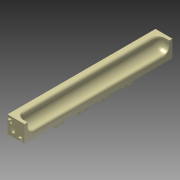
# Autodesk Inventor part: Pillar2
Saved by Autodesk Inventor 2015 (Build 190159000, 159)
## iProperties
Created: 2015-04-20
Part Number: Pillar2
Material: NylonD2W
Document SubType Name: Modeling
Designer: Akovo_000
Density: 1.13 g/cm^3
Appearance: Nylon 6
Mass: 21.3766 g
Surface Area: 162.248 cm^2
Volume: 18.9174 cm^3
Author: Akovo_000
Autodesk Inventor part; units mm, degrees
ref_plane "YZ Plane" through (0, 0, 0) normal (1, 0, 0) x (0, 1, 0)
ref_plane "XZ Plane" through (0, 0, 0) normal (0, 1, 0) x (-1, 0, 0)
ref_plane "XY Plane" through (0, 0, 0) normal (0, 0, 1) x (1, 0, 0)
sketch "Sketch1" plane through (0, 0, 0) normal (0, 1, 0) x (-1, 0, 0)
  line L0 (16, 16) -> (7.6667, 16)
  line L1 (0, 16) -> (0, 8.3333)
  line L2 (16, 16) -> (16, 14)
  line L3 (16, 14) -> (12, 14)
  line L4 (16, 12) -> (16, 7.6667)
  line L5 (0, 0) -> (2, 0)
  line L6 (2, 0) -> (2, 4)
  line L7 (2, 4) -> (4, 4)
  line L8 (4, 0) -> (8.3333, 0)
  circle A0 centre (11, 5) radius 2
  line L9 (12, 10) -> (14, 10)
  line L10 (14, 10) -> (14, 12)
  line L11 (14, 12) -> (16, 12)
  line L12 (12, 10) -> (12, 12)
  line L13 (4, 0) -> (4, 2)
  line L14 (4, 2) -> (6, 2)
  line L15 (6, 2) -> (6, 4)
  line L16 (4, 4) -> (6, 4)
  line L17 (12, 12) -> (12, 14)
  line L18 (7.6667, 16) -> (0, 16)
  line L19 (0, 8.3333) -> (0, 0)
  line L20 (8.3333, 0) -> (16, 0)
  line L21 (16, 7.6667) -> (16, 0)
  line L22 (11, 5) -> (16, 5) construction
  line L23 (11, 5) -> (11, 0) construction
  line L24 (16, 10) -> (6, 10) construction
  line L25 (6, 0) -> (6, 10) construction
  line L26 (6, 10) -> (0, 10) construction
  line L27 (6, 10) -> (6, 16) construction
  line L28 (11, 5) -> (11, 10) construction
  line L29 (11, 5) -> (6, 5) construction
  dimension "d0" = 2
  dimension "d3" = 2
  dimension "d7" = 4
  dimension "d13" = 2
  dimension "d85" = 4
  dimension "d91" = 16
  dimension "d115" = 0
  dimension "d116" = 5
  constraints: 60 end point, 17 perpendicular, 14 equal length, 7 point on line, 6 horizontal, 6 vertical, 4 collinear, 2 midpoint, 1 centre point, 1 parallel
  measures "d0" distance of L2.end L4.start
  measures "d3" distance between parallel lines of L3 L0
  measures "d7" diameter of A0
  measures "d13" distance of L9.start L12.end
  measures "d85" distance of L3.end L2.end
  measures "d91" distance of L0.start L20.end
  measures "d115" distance between parallel lines of L25 L15
  measures "d116" distance from line of L22.start L15
extrude "Attachment Bas" add sketch "Sketch1" along normal blind 3
sketch "Sketch9" plane through (0, 3, 0) normal (0, 1, 0) x (1, 0, 0)
  line L0 (-16, -14) -> (-12, -14)
  line L1 (-12, -14) -> (-12, -10)
  line L2 (-12, -10) -> (-14, -10)
  line L3 (-14, -10) -> (-12, -10) projected
  line L4 (-14, -10) -> (-14, -12)
  line L5 (-14, -12) -> (-16, -12)
  line L6 (-16, -12) -> (-14, -12) projected
  line L7 (-16, -12) -> (-16, -5)
  line L8 (-16, 0) -> (-16, -12) projected
  line L9 (-16, 0) -> (-11, 0) construction
  line L10 (-4, 0) -> (-4, -2)
  line L11 (-4, -2) -> (-6, -2)
  line L12 (-6, -2) -> (-6, -4)
  line L13 (-6, -4) -> (-6, -2) projected
  line L14 (-6, -4) -> (-2, -4)
  line L15 (-2, -4) -> (-2, 0)
  line L16 (-2, 0) -> (-2, -4) projected
  line L17 (-2, 0) -> (0, 0)
  line L18 (0, 0) -> (-2, 0) projected
  line L19 (0, 0) -> (0, -4)
  line L20 (0, -16) -> (-12, -16) construction
  line L21 (-16, -16) -> (-16, -14)
  line L22 (-12, -14) -> (-16, -14) projected
  circle A0 centre (-11, -5) radius 2 projected
  arc A1 (-11, 0) -> (-16, -5) centre (-11, -5) ccw
  line L23 (-4, 0) -> (-16, 0) construction
  line L24 (-16, -5) -> (-16, 0) construction
  line L25 (-11, 0) -> (-4, 0)
  line L26 (-12, -16) -> (-16, -16)
  line L27 (0, -4) -> (0, -16) construction
  line L28 (0, -16) -> (0, 0) projected
  line L29 (-2, -4) -> (-6, -4) projected
  line L30 (-16, -16) -> (0, -16) projected
  circle A2 centre (-11, -5) radius 2 projected
  line L31 (-14.5355, -1.4645) -> (-12.4142, -3.5858) construction
  line L32 (-11, -5) -> (-9.5858, -6.4142) construction
  line L33 (-12, -14) -> (-9, -14) construction
  line L34 (-12, -10) -> (-12, -14) projected
  line L35 (-2, -4) -> (-2, -7) construction
  line L36 (-2, -7) -> (-2, -14) construction
  line L37 (-2, -14) -> (-9.7838, -14) construction
  line L38 (-9.5858, -6.4142) -> (-7.4645, -8.5355) construction
  line L39 (-12.4142, -3.5858) -> (-11, -5) construction
  arc A3 (-7.4645, -8.5355) -> (-9.725, -13.7869) centre (-2, -14) ccw
  arc A4 (-2.2131, -6.275) -> (-7.4645, -8.5355) centre (-2, -14) ccw
  arc A5 (-2.2131, -6.275) -> (0, -4) centre (-2.2759, -4) ccw
  arc A6 (-12, -16) -> (-9.725, -13.7869) centre (-12, -13.7241) ccw
  constraints: 56 end point, 19 perpendicular, 14 collinear, 13 point on circle, 7 tangent, 5 centre point, 5 coincident, 3 equal length, 3 point on line, 2 line through centre, 1 equal radius, 1 horizontal
extrude "curvedpart" add sketch "Sketch9" along normal blind 15 contours L0 L1 L2 L4 L5 L7 A1 L25 L10 L11 L12 L14 L15 L17 L19 A5 A4 A3 A6 L26 L21
sketch "Sketch2" plane through (0, 18, 0) normal (0, 1, 0) x (1, 0, 0)
  line L0 (0, 0) -> (-2, 0)
  line L1 (0, 0) -> (-2, 0) projected
  line L2 (-2, 0) -> (-2, -4)
  line L3 (-2, 0) -> (-2, -4) projected
  line L4 (-2, -4) -> (-6, -4)
  line L5 (-2, -4) -> (-6, -4) projected
  line L6 (-6, -4) -> (-6, -2)
  line L7 (-6, -4) -> (-6, -2) projected
  line L8 (-6, -2) -> (-4, -2)
  line L9 (-6, -2) -> (-4, -2) projected
  line L10 (-4, -2) -> (-4, 0)
  line L11 (-4, -2) -> (-4, 0) projected
  arc A0 (-11, 0) -> (-16, -5) centre (-11, -5) ccw projected
  arc A1 (-11, 0) -> (-16, -5) centre (-11, -5) ccw
  line L12 (-16, -5) -> (-16, -12)
  line L13 (-16, -12) -> (-14, -12)
  line L14 (-16, -12) -> (-14, -12) projected
  line L15 (-12, -10) -> (-12, -14)
  line L16 (-12, -14) -> (-16, -14)
  line L17 (-16, -14) -> (-16, -16)
  line L18 (0, -16) -> (0, 0) projected
  line L19 (-6, -4) -> (-12, -10) construction
  line L20 (-12, -10) -> (-14, -10)
  line L21 (-14, -11) -> (-12, -11) projected
  line L22 (-14, -10) -> (-14, -12)
  line L23 (-14, -12) -> (-14, -10) projected
  line L24 (0, 0) -> (0, -4)
  line L25 (-4, 0) -> (-11, 0)
  line L26 (-4, 0) -> (-16, 0) projected
  line L27 (-9.954, -1.0963) -> (-7.0963, -3.954)
  line L28 (-7.0963, -3.954) -> (-8.1423, -7.8577)
  line L29 (-8.1423, -7.8577) -> (-12.046, -8.9037)
  line L30 (-12.046, -8.9037) -> (-14.9037, -6.046)
  line L31 (-14.9037, -6.046) -> (-13.8577, -2.1423)
  line L32 (-13.8577, -2.1423) -> (-9.954, -1.0963)
  arc A2 (-2.2131, -6.275) -> (-9.725, -13.7869) centre (-2, -14) ccw
  arc A3 (-2.2131, -6.275) -> (0, -4) centre (-2.2759, -4) ccw
  arc A4 (-12, -16) -> (-9.725, -13.7869) centre (-12, -13.7241) ccw
  line L33 (-12, -16) -> (-16, -16)
  line L34 (-16, -16) -> (0, -16) projected
  dimension "d103" = 7
  constraints: 46 end point, 10 collinear, 8 point on circle, 4 centre point, 3 perpendicular, 3 tangent, 3 vertical, 2 coincident, 1 parallel, 13 other
  measures "d103" distance between parallel lines of L27 L30
extrude "BossForNut" add sketch "Sketch2" along normal blind 3 contours L18 A3 A2 A4 L33 L17 L16 L15 L20 L22 L13 L12 A0 L25 L10 L8 L6 L4 L2 L0
sketch "Sketch3" plane through (0, 21, 0) normal (0, 1, 0) x (1, 0, 0)
  line L0 (-16, -5) -> (-16, -6.9497)
  arc A0 (-11, 0) -> (-16, -5) centre (-11, -5) ccw projected
  line L1 (-16, -5) -> (-16, -12) projected
  line L2 (-16, -12) -> (-14, -12)
  line L3 (-14, -12) -> (-14, -10)
  line L4 (-14, -12) -> (-14, -10) projected
  line L5 (-14, -10) -> (-12, -10)
  line L6 (-12, -10) -> (-12, -14)
  line L7 (-12, -14) -> (-16, -14)
  line L8 (-16, -14) -> (-16, -16) projected
  line L9 (-16, -14) -> (-16, -16)
  arc A1 (-11, 0) -> (-11.05, -0.0003) centre (-11, -5) ccw
  line L10 (0, -4) -> (0, 0)
  line L11 (0, -4) -> (0, 0) projected
  line L12 (0, 0) -> (-2, 0)
  line L13 (0, 0) -> (-2, 0) projected
  line L14 (-2, 0) -> (-2, -4)
  line L15 (-2, -4) -> (-6, -4)
  line L16 (-2, -4) -> (-6, -4) projected
  line L17 (-6, -4) -> (-6, -2)
  line L18 (-6, -2) -> (-4, -2)
  line L19 (-6, -2) -> (-4, -2) projected
  line L20 (-4, -2) -> (-4, 0)
  line L21 (-4, 0) -> (-11, 0)
  line L22 (-4, 0) -> (-11, 0) projected
  line L23 (-8.1423, -7.8577) -> (-12.046, -8.9037)
  line L24 (-12.046, -8.9037) -> (-8.1423, -7.8577) projected
  line L25 (-12.046, -8.9037) -> (-14.9037, -6.046)
  line L26 (-14.9037, -6.046) -> (-13.8577, -2.1423) construction
  line L27 (-14.9037, -6.046) -> (-13.8577, -2.1423) projected
  line L28 (-13.8577, -2.1423) -> (-9.954, -1.0963) construction
  line L29 (-13.8577, -2.1423) -> (-9.954, -1.0963) construction
  line L30 (-9.954, -1.0963) -> (-7.0963, -3.954)
  line L31 (-7.0963, -3.954) -> (-8.1423, -7.8577)
  line L32 (-12.046, -8.9037) -> (-14.9037, -6.046) projected
  line L33 (-9.954, -1.0963) -> (-7.0963, -3.954) projected
  arc A2 (-2.2131, -6.275) -> (0, -4) centre (-2.2759, -4) ccw
  line L34 (-12, -16) -> (-16, -16)
  line L35 (-16, -16) -> (-12, -16) projected
  arc A3 (-12, -16) -> (-9.725, -13.7869) centre (-12, -13.7241) ccw
  arc A4 (-2.2131, -6.275) -> (-9.725, -13.7869) centre (-2, -14) ccw
  line L36 (-9.954, -1.0963) -> (-11.05, -0.0003)
  line L37 (-14.9037, -6.046) -> (-15.9997, -4.95)
  arc A5 (-15.9997, -4.95) -> (-16, -5) centre (-11, -5) ccw
  arc A6 (-11.05, -0.0003) -> (-15.9997, -4.95) centre (-11, -5) ccw construction
  line L38 (-16, -6.9497) -> (-16, -12)
  point P0 (-9.0503, 0)
  constraints: 50 end point, 15 collinear, 15 point on circle, 8 perpendicular, 6 centre point, 6 tangent, 2 parallel, 2 point on line, 1 coincident
extrude "NutInserter" add sketch "Sketch3" along normal blind 5 contours A0 L37 L25 L23 L31 L30 L36 L21 L20 L18 L17 L15 L14 L12 L10 A2 A4 A3 L34 L8 L7 L6 L5 L3 L2 L1 L0
sketch "Sketch4" plane through (0, 26, 0) normal (0, 1, 0) x (1, 0, 0)
  line L0 (-12, -10) -> (-14, -10)
  line L1 (-14, -10) -> (-12, -10) projected
  line L2 (-14, -10) -> (-14, -12)
  line L3 (-14, -12) -> (-14, -10) projected
  line L4 (-14, -12) -> (-16, -12)
  line L5 (-16, -12) -> (-14, -12) projected
  line L6 (-16, -12) -> (-16, -5)
  line L7 (-16, -5) -> (-16, -12) projected
  line L8 (-12, -10) -> (-12, -14)
  line L9 (-12, -14) -> (-16, -14)
  line L10 (-16, -14) -> (-16, -16)
  line L11 (-16, -14) -> (-16, -16) projected
  line L12 (-16, -16) -> (-12, -16)
  line L13 (-11, 0) -> (-4, 0)
  line L14 (-4, 0) -> (-11, 0) projected
  line L15 (-4, 0) -> (-4, -2)
  line L16 (-4, -2) -> (-6, -2)
  line L17 (-6, -2) -> (-4, -2) projected
  line L18 (-6, -2) -> (-6, -4)
  line L19 (-6, -4) -> (-2, -4)
  line L20 (-2, -4) -> (-6, -4) projected
  line L21 (-2, -4) -> (-2, 0)
  line L22 (-2, 0) -> (0, 0)
  line L23 (0, 0) -> (-2, 0) projected
  line L24 (0, 0) -> (0, -4)
  arc A0 (-11, 0) -> (-16, -5) centre (-11, -5) ccw
  arc A1 (-2.2131, -6.275) -> (0, -4) centre (-2.2759, -4) ccw
  arc A2 (-2.2131, -6.275) -> (-9.725, -13.7869) centre (-2, -14) ccw
  arc A3 (-12, -16) -> (-9.725, -13.7869) centre (-12, -13.7241) ccw
  circle A4 centre (-11, -5) radius 3
  point P0 (-11.5, -5.5)
  dimension "d130" = 6
  constraints: 32 end point, 9 collinear, 8 point on circle, 6 perpendicular, 5 centre point, 4 tangent, 1 coincident, 1 point on line, 1 vertical
  measures "d130" diameter of A4
extrude "Main Pillar" add sketch "Sketch4" along normal blind 88
sketch "Sketch5" plane through (0, 114, 0) normal (0, 1, 0) x (1, 0, 0)
  line L0 (-2, 0) -> (-2, -4)
  line L1 (-2, -4) -> (-6, -4)
  line L2 (-2, -4) -> (-6, -4) projected
  line L3 (-6, -4) -> (-6, -2)
  line L4 (-6, -2) -> (-4, -2)
  line L5 (-6, -2) -> (-4, -2) projected
  line L6 (-4, -2) -> (-4, 0)
  line L7 (-4, -2) -> (-4, 0) projected
  line L8 (-4, 0) -> (-11, 0)
  line L9 (-4, 0) -> (-16, 0) projected
  line L10 (-16, -5) -> (-16, -12)
  line L11 (-16, -12) -> (-14, -12)
  line L12 (-14, -12) -> (-14, -10)
  line L13 (-14, -12) -> (-14, -10) projected
  line L14 (-14, -10) -> (-12, -10)
  line L15 (-14, -10) -> (-12, -10) projected
  line L16 (-12, -10) -> (-12, -14)
  line L17 (-12, -14) -> (-16, -14)
  line L18 (-12, -14) -> (-16, -14) projected
  line L19 (-16, -14) -> (-16, -16)
  line L20 (-16, -16) -> (-12, -16)
  line L21 (-16, -16) -> (-12, -16) projected
  line L22 (-2, 0) -> (0, 0)
  line L23 (0, 0) -> (-2, 0) projected
  line L24 (0, 0) -> (0, -4)
  arc A0 (-11, 0) -> (-11.05, -0.0003) centre (-11, -5) ccw
  arc A1 (-2.2131, -6.275) -> (0, -4) centre (-2.2759, -4) ccw
  arc A2 (-12, -16) -> (-9.725, -13.7869) centre (-12, -13.7241) ccw
  arc A3 (-2.2131, -6.275) -> (-9.725, -13.7869) centre (-2, -14) ccw
  line L25 (-12.046, -8.9037) -> (-14.9037, -6.046)
  line L26 (-14.9037, -6.046) -> (-13.8577, -2.1423) construction
  line L27 (-13.8577, -2.1423) -> (-9.954, -1.0963) construction
  line L28 (-9.954, -1.0963) -> (-7.0963, -3.954)
  line L29 (-7.0963, -3.954) -> (-8.1423, -7.8577)
  line L30 (-8.1423, -7.8577) -> (-12.046, -8.9037)
  line L31 (-9.954, -1.0963) -> (-11.05, -0.0003)
  line L32 (-14.9037, -6.046) -> (-15.9997, -4.95)
  line L33 (-15.9997, -4.95) -> (-14.9037, -6.046) projected
  arc A4 (-15.9997, -4.95) -> (-16, -5) centre (-11, -5) ccw
  arc A5 (-11.05, -0.0003) -> (-15.9997, -4.95) centre (-11, -5) ccw construction
  constraints: 49 end point, 12 point on circle, 10 collinear, 6 centre point, 6 tangent, 5 perpendicular, 2 vertical, 1 coincident, 13 other
extrude "NutInserter2" add sketch "Sketch5" along normal blind 5
sketch "Sketch6" plane through (0, 119, 0) normal (0, 1, 0) x (1, 0, 0)
  circle A0 centre (-11, -5) radius 2 projected
  line L0 (-14.9037, -6.046) -> (-13.8577, -2.1423)
  line L1 (-13.8577, -2.1423) -> (-9.954, -1.0963)
  line L2 (-9.954, -1.0963) -> (-7.0963, -3.954)
  line L3 (-7.0963, -3.954) -> (-8.1423, -7.8577)
  line L4 (-8.1423, -7.8577) -> (-12.046, -8.9037)
  line L5 (-12.046, -8.9037) -> (-14.9037, -6.046)
  line L6 (-16, -12) -> (-14, -12)
  line L7 (-16, -12) -> (-14, -12) projected
  line L8 (-14, -12) -> (-14, -10)
  line L9 (-14, -12) -> (-14, -10) projected
  line L10 (-14, -10) -> (-12, -10)
  line L11 (-14, -10) -> (-12, -10) projected
  line L12 (-12, -10) -> (-12, -14)
  line L13 (-12, -10) -> (-12, -14) projected
  line L14 (-12, -14) -> (-16, -14)
  line L15 (-16, -14) -> (-16, -16)
  line L16 (-16, -14) -> (-16, -16) projected
  line L17 (-16, -16) -> (-12, -16)
  line L18 (0, 0) -> (0, -4)
  line L19 (0, -4) -> (0, 0) projected
  line L20 (0, 0) -> (-2, 0)
  line L21 (-2, 0) -> (-2, -4) projected
  line L22 (-2, 0) -> (-2, -4)
  line L23 (-2, -4) -> (-6, -4)
  line L24 (-2, -4) -> (-6, -4) projected
  line L25 (-6, -4) -> (-6, -2)
  line L26 (-6, -4) -> (-6, -2) projected
  line L27 (-6, -2) -> (-4, -2)
  line L28 (-4, -2) -> (-4, 0)
  line L29 (-4, 0) -> (-11, 0)
  line L30 (-4, 0) -> (-11, 0) projected
  line L31 (-16, -12) -> (-16, -5)
  arc A1 (-11, 0) -> (-16, -5) centre (-11, -5) ccw
  arc A2 (-12, -16) -> (-9.725, -13.7869) centre (-12, -13.7241) ccw
  arc A3 (-2.2131, -6.275) -> (-9.725, -13.7869) centre (-2, -14) ccw
  arc A4 (-2.2131, -6.275) -> (0, -4) centre (-2.2759, -4) ccw
  point P0 (-11, -5)
  constraints: 44 end point, 10 collinear, 8 point on circle, 6 tangent, 5 perpendicular, 4 centre point, 1 coincident, 1 vertical, 13 other
extrude "BossFotNut2" add sketch "Sketch6" along normal blind 3 contours L31 A1 L29 L28 L27 L25 L23 L21 L20 L18 A4 A3 A2 L17 L15 L14 L12 L10 L8 L6
sketch "Sketch10" plane through (0, 122, 0) normal (0, 1, 0) x (1, 0, 0)
  line L0 (-12, -14) -> (-16, -14) projected
  line L1 (-12, -14) -> (-12, -10)
  line L2 (-12, -10) -> (-12, -14) projected
  line L3 (-12, -10) -> (-14, -10)
  line L4 (-14, -10) -> (-14, -12)
  line L5 (-14, -12) -> (-14, -10) projected
  line L6 (-16, -12) -> (-14, -12) projected
  line L7 (-16, -14) -> (-16, -16)
  line L8 (-16, -16) -> (-12, -16)
  line L9 (-16, -16) -> (-12, -16) projected
  line L10 (0, -4) -> (0, 0)
  line L11 (0, -4) -> (0, 0) projected
  line L12 (0, 0) -> (-2, 0)
  line L13 (-2, 0) -> (-2, -4)
  line L14 (-2, -4) -> (-6, -4)
  line L15 (-2, -4) -> (-6, -4) projected
  line L16 (-6, -4) -> (-6, -2)
  line L17 (-6, -4) -> (-6, -2) projected
  line L18 (-6, -2) -> (-4, -2)
  line L19 (-6, -2) -> (-4, -2) projected
  line L20 (-4, -2) -> (-4, 0)
  arc A0 (-2.2131, -6.275) -> (0, -4) centre (-2.2759, -4) ccw
  arc A1 (-2.2131, -6.275) -> (-9.725, -13.7869) centre (-2, -14) ccw
  arc A2 (-12, -16) -> (-9.725, -13.7869) centre (-12, -13.7241) ccw
  circle A3 centre (-11, -5) radius 2 projected
  circle A4 centre (-11, -5) radius 2
  line L21 (-14, -12) -> (-16, -12)
  line L22 (-12, -14) -> (-16, -14)
  line L23 (-16, -12) -> (-16, -5)
  line L24 (-16, -5) -> (-16, -12) projected
  line L25 (-4, 0) -> (-11, 0)
  line L26 (-11, 0) -> (-16, 0) projected
  arc A5 (-11, 0) -> (-16, -5) centre (-11, -5) ccw
  constraints: 32 end point, 10 collinear, 8 point on circle, 5 centre point, 5 tangent, 4 perpendicular, 1 coincident, 1 horizontal, 1 vertical
extrude "CurvedTransition" add sketch "Sketch10" along normal blind 15
sketch "Sketch7" plane through (0, 137, 0) normal (0, 1, 0) x (1, 0, 0)
  line L0 (0, -16) -> (-16, -16)
  line L1 (-16, -16) -> (-11.1769, -16)
  line L2 (-16, -16) -> (-16, -14)
  line L3 (-16, -14) -> (-16, -16)
  line L4 (-16, -14) -> (-12, -14)
  line L5 (-12, -14) -> (-16, -14)
  line L6 (-12, -14) -> (-12, -10)
  line L7 (-12, -10) -> (-14, -10)
  line L8 (-14, -10) -> (-14, -12)
  line L9 (-14, -12) -> (-16, -12)
  line L10 (-16, -12) -> (-14, -12)
  line L11 (-16, -12) -> (-16, 0)
  line L12 (-16, 0) -> (-16, -5.5)
  circle A0 centre (-11, -5) radius 2
  circle A1 centre (-11, -5) radius 2
  line L13 (-16, 0) -> (-16, -5) projected
  line L14 (-12, -16) -> (0, -16) projected
  line L15 (-16, -14) -> (-16, -16) projected
  line L16 (-12, -14) -> (-16, -14) projected
  line L17 (-12, -10) -> (-12, -14) projected
  line L18 (-14, -10) -> (-12, -10) projected
  line L19 (-14, -12) -> (-14, -10) projected
  line L20 (-16, -12) -> (-14, -12) projected
  circle A2 centre (-11, -5) radius 2 projected
  line L21 (-2, 0) -> (-2, -4) projected
  line L22 (-16, 0) -> (-4, 0)
  line L23 (-4, 0) -> (-16, 0) projected
  line L24 (-4, 0) -> (-4, -2)
  line L25 (-4, -2) -> (-4, 0) projected
  line L26 (-4, -2) -> (-6, -2)
  line L27 (-6, -2) -> (-6, -4)
  line L28 (-6, -4) -> (-6, -2) projected
  line L29 (-6, -4) -> (-2, -4)
  line L30 (-2, -4) -> (-2, 0)
  line L31 (-2, 0) -> (0, 0)
  line L32 (0, 0) -> (-2, 0) projected
  line L33 (0, -16) -> (0, 0)
  line L34 (0, -16) -> (0, 0) projected
  constraints: 42 end point, 19 collinear, 4 perpendicular, 2 centre point, 1 coincident, 1 concentric, 1 horizontal
extrude "Attachment Base 2" add sketch "Sketch7" along normal blind 3
fillet "Fillet2" radius 6 6 edges at (-7.4645, 3, 8.5355) (-10.4131, 3, 15.3554) (-0.6446, 3, 5.5869) (-0.6446, 137, 5.5869) (-10.4131, 137, 15.3554) (-7.4645, 137, 8.5355)
fillet "Fillet2" radius 2 2 edges at (-14.5355, 137, 1.4645) (-14.5355, 3, 1.4645)
sketch "Sketch12" plane through (-4, 0, 0) normal (1, 0, 0) x (0, 0, -1)
  line L0 (6.1, 140) -> (6.1, 120) construction
  line L1 (6.1, 0) -> (0, 0) construction
  line L2 (6.1, 120) -> (0, 120) construction
  line L3 (6.1, 107.2) -> (3, 107.2)
  line L4 (6.1, 98.2) -> (3, 98.2)
  line L5 (0, 0) -> (0, 140) projected
  line L6 (0, 120) -> (0, 110.2)
  line L7 (0, 107.2) -> (0, 105.25)
  line L8 (0, 95.2) -> (0, 88.4)
  line L9 (6.1, 63.6) -> (3, 63.6)
  line L10 (0, 5) -> (0, 135) projected
  line L11 (6.1, 54.6) -> (3, 54.6)
  line L12 (6.1, 41.8) -> (3, 41.8)
  line L13 (6.1, 32.8) -> (3, 32.8)
  line L14 (6.1, 20) -> (0, 20) construction
  line L15 (6.1, 120) -> (6.1, 107.2) construction
  line L16 (6.1, 107.2) -> (6.1, 105.25)
  line L17 (6.1, 98.2) -> (6.1, 85.4) construction
  line L18 (6.1, 63.6) -> (6.1, 61.65)
  line L19 (6.1, 41.8) -> (6.1, 39.85)
  line L20 (6.1, 32.8) -> (6.1, 20) construction
  line L21 (6.1, 54.6) -> (6.1, 41.8) construction
  line L22 (6.1, 20) -> (6.1, 0) construction
  line L23 (0, 20) -> (0, 0)
  line L24 (0, 29.8) -> (0, 20)
  line L25 (0, 41.8) -> (0, 39.85)
  line L26 (0, 51.6) -> (0, 44.8)
  line L27 (0, 63.6) -> (0, 61.65)
  line L28 (6.1, 85.4) -> (3, 85.4)
  line L29 (6.1, 76.4) -> (3, 76.4)
  line L30 (6.1, 85.4) -> (6.1, 83.45)
  line L31 (0, 73.4) -> (0, 66.6)
  line L32 (0, 85.4) -> (0, 83.45)
  line L33 (6.1, 76.4) -> (6.1, 63.6) construction
  line L34 (6.1, 105.25) -> (3.1, 105.25) construction
  line L35 (6.1, 100.15) -> (3.1, 100.15) construction
  line L36 (6.1, 105.25) -> (6.1, 104)
  line L37 (6.1, 100.15) -> (6.1, 98.2)
  line L38 (6.1, 104) -> (3.1, 104)
  line L39 (3.1, 104) -> (3.1, 105.25)
  line L40 (6.1, 101.4) -> (3.1, 101.4)
  line L41 (3.1, 101.4) -> (3.1, 100.15)
  line L42 (6.1, 101.4) -> (6.1, 100.15)
  line L43 (6.1, 104) -> (6.1, 101.4)
  line L44 (3.1, 100.15) -> (0, 100.15)
  line L45 (3.1, 105.25) -> (0, 105.25)
  line L46 (6.1, 104) -> (6.1, 105.25)
  line L47 (6.1, 101.4) -> (6.1, 100.15)
  line L48 (0, 100.15) -> (0, 98.2)
  line L49 (0, 105.25) -> (0, 100.15)
  arc A0 (0, 110.2) -> (3, 107.2) centre (3, 110.2) ccw
  arc A1 (3, 98.2) -> (0, 95.2) centre (3, 95.2) ccw
  arc A2 (0, 88.4) -> (3, 85.4) centre (3, 88.4) ccw
  arc A3 (3, 76.4) -> (0, 73.4) centre (3, 73.4) ccw
  arc A4 (0, 66.6) -> (3, 63.6) centre (3, 66.6) ccw
  arc A5 (3, 54.6) -> (0, 51.6) centre (3, 51.6) ccw
  arc A6 (0, 44.8) -> (3, 41.8) centre (3, 44.8) ccw
  arc A7 (3, 32.8) -> (0, 29.8) centre (3, 29.8) ccw
  line L50 (6.1, 83.45) -> (3.1, 83.45) construction
  line L51 (0, 78.35) -> (3.1, 78.35)
  line L52 (6.1, 82.2) -> (3.1, 82.2)
  line L53 (3.1, 82.2) -> (3.1, 83.45)
  line L54 (6.1, 79.6) -> (3.1, 79.6)
  line L55 (3.1, 79.6) -> (3.1, 78.35)
  line L56 (6.1, 82.2) -> (6.1, 79.6)
  line L57 (6.1, 83.45) -> (6.1, 82.2)
  line L58 (6.1, 79.6) -> (6.1, 78.35)
  line L59 (6.1, 78.35) -> (6.1, 76.4)
  line L60 (3.1, 83.45) -> (0, 83.45)
  line L61 (3.1, 78.35) -> (6.1, 78.35) construction
  line L62 (6.1, 61.65) -> (3.1, 61.65) construction
  line L63 (6.1, 56.55) -> (3.1, 56.55) construction
  line L64 (3.1, 56.55) -> (3.1, 57.8)
  line L65 (3.1, 57.8) -> (6.1, 57.8)
  line L66 (6.1, 60.4) -> (3.1, 60.4)
  line L67 (3.1, 60.4) -> (3.1, 61.65)
  line L68 (3.1, 61.65) -> (0, 61.65)
  line L69 (3.1, 56.55) -> (0, 56.55)
  line L70 (6.1, 57.8) -> (6.1, 56.55)
  line L71 (6.1, 60.4) -> (6.1, 57.8)
  line L72 (6.1, 61.65) -> (6.1, 60.4)
  line L73 (6.1, 56.55) -> (6.1, 54.6)
  line L74 (6.1, 39.85) -> (3.1, 39.85) construction
  line L75 (6.1, 34.75) -> (3.1, 34.75) construction
  line L76 (3.1, 39.85) -> (3.1, 38.6)
  line L77 (3.1, 38.6) -> (6.1, 38.6)
  line L78 (6.1, 36) -> (3.1, 36)
  line L79 (3.1, 36) -> (3.1, 34.75)
  line L80 (6.1, 39.85) -> (6.1, 38.6)
  line L81 (6.1, 38.6) -> (6.1, 36)
  line L82 (6.1, 36) -> (6.1, 34.75)
  line L83 (6.1, 34.75) -> (6.1, 32.8)
  line L84 (3.1, 34.75) -> (0, 34.75)
  line L85 (3.1, 39.85) -> (0, 39.85)
  line L86 (0, 83.45) -> (0, 78.35)
  line L87 (0, 78.35) -> (0, 76.4)
  line L88 (0, 61.65) -> (0, 56.55)
  line L89 (0, 56.55) -> (0, 54.6)
  line L90 (0, 39.85) -> (0, 34.75)
  line L91 (0, 34.75) -> (0, 32.8)
  line L92 (0, 32.8) -> (0, 29.8)
  line L93 (0, 41.8) -> (0, 44.8)
  line L94 (0, 51.6) -> (0, 54.6)
  line L95 (0, 63.6) -> (0, 66.6)
  line L96 (0, 73.4) -> (0, 76.4)
  line L97 (0, 88.4) -> (0, 85.4)
  line L98 (0, 95.2) -> (0, 98.2)
  line L99 (0, 0) -> (0, 140) projected
  line L100 (0, 110.2) -> (0, 107.2)
  line L101 (0, 120) -> (0, 140)
  line L102 (6.1, 140) -> (0, 140)
  dimension "d138" = 9
  dimension "d140" = 5.1
  dimension "d141" = 2.6
  dimension "d142" = 3.1
  dimension "d143" = 3
  dimension "d144" = 0
  dimension "d148" = 3
  dimension "d159" = 20
  dimension "d160" = 20
  constraints: 198 end point, 98 perpendicular, 62 point on line, 45 collinear, 21 tangent, 17 point on circle, 13 horizontal, 8 centre point, 7 equal radius, 6 parallel, 4 vertical, 21 other
  measures "d138" distance between parallel lines of L4 L3
  measures "d140" distance between parallel lines of L35 L34
  measures "d141" distance of L36.end L40.start
  measures "d142" distance of the line from the sketch origin of L41
  measures "d143" distance between parallel lines of L47 L41
  measures "d144" distance between parallel lines of L42 L47
  measures "d148" radius of A0
  measures "d159" distance between parallel lines of L1 L14
  measures "d160" distance between parallel lines of L2 L102
extrude "Extrusion14" add sketch "Sketch12" against normal blind 12 contours L16 L36 L38 L39 L45 L5 A0 L3 | L42 L37 L4 A1 L5 L44 L41 L40 | L5 L84 L79 L78 L82 L83 L13 A7 | L5 A6 L12 L19 L80 L77 L76 L85 | L5 L69 L64 L65 L70 L73 L11 A5 | L5 A4 L9 L18 L72 L66 L67 L68 | L5 L51 L55 L54 L58 L59 L29 A3 | L5 A2 L28 L30 L57 L52 L53 L60
sketch "Sketch13" plane through (-16, 0, 0) normal (-1, 0, 0) x (0, 0, 1)
  line L0 (3.4908, 42.8165) -> (3.4908, 46.8807)
  line L1 (0, 44.8) -> (2.5, 44.8)
  line L2 (0, 39.85) -> (0, 44.8)
  line L3 (0, 0) -> (0, 140) projected
  line L4 (0, 34.75) -> (2.5, 34.75)
  line L5 (2.5, 34.75) -> (2.5, 29.8)
  line L6 (2.5, 29.8) -> (0, 29.8)
  line L7 (0, 29.8) -> (0, 34.75)
  line L8 (0, 39.85) -> (2.5, 39.85)
  line L9 (2.5, 39.85) -> (2.5, 44.8)
  line L10 (0, 51.6) -> (2.5, 51.6)
  line L11 (2.5, 51.6) -> (2.5, 56.55)
  line L12 (2.5, 56.55) -> (0, 56.55)
  line L13 (0, 51.6) -> (0, 56.55)
  line L14 (0, 61.65) -> (2.5, 61.65)
  line L15 (2.5, 61.65) -> (2.5, 72.6542)
  line L16 (0, 73.4) -> (2, 73.4)
  line L17 (2, 0) -> (2, 140) projected
  line L18 (0, 78.35) -> (2, 78.35)
  line L19 (-3.1, 78.35) -> (0, 78.35) projected
  line L20 (2, 73.4) -> (2, 78.35)
  line L21 (0, 83.45) -> (2, 83.45)
  line L22 (0, 88.4) -> (2, 88.4)
  line L23 (2, 83.45) -> (2, 88.4)
  line L24 (0, 88.4) -> (0, 83.45)
  arc A0 (-3, 85.4) -> (0, 88.4) centre (-3, 88.4) ccw projected
  line L25 (0, 78.35) -> (0, 73.4)
  line L26 (0, 95.2) -> (2, 95.2)
  line L27 (0, 100.15) -> (2, 100.15)
  line L28 (2, 95.2) -> (2, 100.15)
  line L29 (0, 105.25) -> (2, 105.25)
  line L30 (0, 110.2) -> (2, 110.2)
  line L31 (2, 110.2) -> (2, 105.25)
  line L32 (0, 105.25) -> (0, 110.2)
  arc A1 (-3, 107.2) -> (0, 110.2) centre (-3, 110.2) ccw projected
  line L33 (0, 100.15) -> (0, 95.2)
  arc A2 (0, 95.2) -> (-3, 98.2) centre (-3, 95.2) ccw projected
  line L34 (0, 72.6542) -> (2.5, 72.6542)
  line L35 (0, 72.6542) -> (0, 61.65)
  point P0 (0, 150)
  point P1 (2.5, 150)
  point P2 (0, 147)
  point P3 (2.5, 147)
  dimension "d149" = 2.5
  dimension "d161" = 140
  constraints: 66 end point, 13 vertical, 12 horizontal, 5 parallel, 4 perpendicular, 3 tangent, 1 collinear, 11 other
  measures "d149" distance between parallel lines of L5 L7
  measures "d161" distance of point (0, 140) point (0, 0)
extrude "Extrusion15" add sketch "Sketch13" against normal blind 4.5 contours L1 L17 L8 L2 | L1 L9 L8 L17 | L3 L12 L17 L10 | L17 L12 L11 L10 | L4 L17 L6 L3 | L4 L5 L6 L17 | L3 L34 L17 L14 | L17 L34 L15 L14 | L3 L18 L17 L16 | L3 L22 L17 L21 | L3 L27 L17 L26 | L3 L30 L17 L29
body "Solid1"
